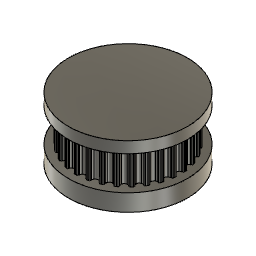
GT2 Pulley (parametric) v4 (Autodesk Fusion 360 design; units mm, degrees)
Autodesk Fusion 360 part; units mm, degrees
sketch "tooth profile" plane through (0, 0, 0) normal (0, 0, 1) x (1, 0, 0)
  circle A0 centre (0, 0) radius 9.5493 construction
  circle A1 centre (0, 0) radius 9.2953 construction
  circle A2 centre (0, 0) radius 8.5453 construction
  line L0 (0, 0) -> (0, 9.3781) construction
  line L1 (0, 0) -> (0.9895, 9.414) construction
  line L2 (0, 0) -> (1.4012, 9.4892) construction
  arc A3 (0.5539, 8.6629) -> (0.8932, 8.4985) centre (0.9512, 9.0504) ccw
  arc A4 (0.3589, 9.1498) -> (0.3788, 8.9921) centre (1.3579, 9.1956) ccw
  circle A5 centre (0, 0) radius 9.1453 construction
  arc A6 (0.3589, 9.1498) -> (0.2092, 9.2929) centre (0.2091, 9.1429) ccw
  arc A7 (0.3788, 8.9921) -> (0.5539, 8.6629) centre (1.0302, 9.1275) ccw
  arc A8 (-0.2092, 9.2929) -> (-0.3589, 9.1498) centre (-0.2091, 9.1429) ccw
  arc A9 (-0.3788, 8.9921) -> (-0.3589, 9.1498) centre (-1.3579, 9.1956) ccw
  arc A10 (-0.5539, 8.6629) -> (-0.3788, 8.9921) centre (-1.0302, 9.1275) ccw
  arc A11 (-0.8932, 8.4985) -> (-0.5539, 8.6629) centre (-0.9512, 9.0504) ccw
  arc A12 (0.8932, 8.4985) -> (-0.8932, 8.4985) centre (0, 0) ccw
  line L3 (0, 9.2953) -> (0.2092, 9.2929)
  line L4 (0, 9.2953) -> (-0.2092, 9.2929)
  circle A13 centre (0, 0) radius 8.5453
  dimension "d35" = 6
  dimension "d36" = 2.4
  dimension "d37" = 0.75
  dimension "d38" = 1.004
  dimension "d40" = 0.15
  dimension "d41" = 0.15
  dimension "d42" = 1
  dimension "d43" = 0.555
  dimension "d68" = 0.2092
  dimension "d69" = 0.6654
  dimension "d88" = 17.0906
  dimension "d89" = 17.0906
  constraint coincident A0.centre A1.centre
  constraint vertical L0
  constraint coincident A1 A4.centre
  constraint coincident L2 A4.centre
  constraint concentric A0 A5
  constraint coincident A5 A6.centre
  constraint tangent A2 A3
  constraint coincident L1 A3.centre
  constraint coincident A4.start A6.start
  constraint coincident A2 A3.end
  constraint tangent A3 A7
  constraint tangent A4 A7
  constraint symmetric L0 A3.start A10.start
  constraint symmetric L0 A3.end A11.start
  constraint symmetric L0 A3 A11
  constraint symmetric L0 A4.start A8.end
  constraint symmetric L0 A4.end A9.start
  constraint symmetric L0 A4 A9
  constraint symmetric L0 A6.end A8.start
  constraint symmetric L0 A6 A8
  constraint symmetric L0 A7 A10
  constraint tangent A4 A6
  constraint coincident L0 L3.start
  constraint coincident A1 L3.start
  constraint symmetric L0 L3.start L4.start
  constraint concentric A0 A13
  measures "d35" angle of L0 L1
  measures "d36" angle of L1 L2
  measures "d37" distance of A1 A2
  measures "d38" distance of A0 A2
  measures "d40" distance of A1 A5
  measures "d41" radius of A6
  measures "d42" radius of A4
  measures "d43" radius of A3
  measures "d68" horizontal distance of L3.start A8.start
  measures "d69" radius of A7
  measures "d88" diameter of A13
  measures "d89" diameter of A13
sketch "left flange" plane through (0, 0, 0) normal (0, 0, 1) x (1, 0, 0)
  circle A0 centre (0, 0) radius 10.5493
  dimension "d44" = 21.0986
  constraint coincident A0.centre origin
  measures "d44" diameter of A0
extrude "Extrude1" add sketch "left flange" along normal blind 11 makes body 1
extrude "Extrude2" cut sketch "left flange" along normal blind 9 bodies 1
ref_plane "WorkPlane2" through (0, 0, -2) normal (0, 0, 1) x (1, 0, 0)
sketch "right flange" plane through (0, 0, -2) normal (0, 0, 1) x (1, 0, 0)
  circle A0 centre (0, 0) radius 10.5493
  dimension "d75" = 21.0986
  constraint coincident A0.centre origin
  measures "d75" diameter of A0
extrude "Extrude11" add sketch "right flange" along normal blind 11 separate body makes body 2
extrude "Extrude12" cut 1 faces at (-1.6728, 1.987, 9) along direction (0, 0, -1) blind 6 on bodies 2 bodies 2
extrude "Extrude13" cut 1 faces at (-1.6728, 1.987, -2) along direction (0, 0, 1) blind 2 on bodies 2 bodies 2
extrude "Extrude14" add sketch "tooth profile" along normal blind 9 separate body contours A3 A4 A6 A7 A8 A9 A10 A11 A12 L3 L4 A13 makes body 3
pattern_circular "C-Pattern2" count 30 over 360 about axis through (0, 0, 1.75) along (0, 0, 1) of bodies 3 makes body 4 at (-1.0907, 8.4754, 3) makes body 5 at (-4.0993, 7.4979, 6) makes body 6 at (-5.5686, 6.4817, 6) makes body 7 at (-6.7945, 5.1823, 6) makes body 8 at (-7.4497, 4.1863, 6) makes body 9 at (-7.8853, 3.2931, 3) makes body 10 at (-8.3976, 1.5817, 3) makes body 11 at (-8.543, -0.1988, 3) makes body 12 at (-8.0958, -2.735, 6) makes body 13 at (-7.7235, -3.6564, 3) makes body 14 at (-6.7945, -5.1823, 3) makes body 15 at (-5.5686, -6.4817, 3) makes body 16 at (-4.0993, -7.4979, 3) makes body 17 at (-2.4508, -8.1863, 3) makes body 18 at (-0.6952, -8.517, 3) makes body 19 at (1.8738, -8.3373, 6) makes body 20 at (4.0993, -7.4979, 6) makes body 21 at (4.4437, -7.299, 3) makes body 22 at (6.4165, -5.6436, 6) makes body 23 at (7.0283, -4.8606, 3) makes body 24 at (7.8853, -3.2931, 3) makes body 25 at (8.3976, -1.5817, 3) makes body 26 at (8.543, 0.1988, 3) makes body 27 at (7.8853, 3.2931, 6) makes body 28 at (7.7235, 3.6564, 3) makes body 29 at (6.7945, 5.1823, 3) makes body 30 at (5.5686, 6.4817, 3) makes body 31 at (4.0993, 7.4979, 3) makes body 32 at (2.4508, 8.1863, 3)
extrude "Extrude16" add sketch "tooth profile" along normal blind 9 contours A12 A13 bodies 2 23 24 25 26 27 28 29 30 31 32 3 1 4 5 6 7 8 9 10 11 12 13 14 15 16 17 18 19 20 21 22
equation "pitch = 2 mm"
equation "shoulder_radius = 0.15 mm"
equation "transition_radius = 1.0 mm"
equation "tooth_radius = 0.555 mm"
equation "b = 0.4 mm"
equation "tooth_height = 0.75 mm"
equation "pld_to_tooth_root = 0.254 mm"
equation "flange_width_left = 2 mm"
equation "flange_height_left = 2 mm"
equation "flange_width_right = 3 mm"
equation "flange_height_right = 2 mm"
equation "tooth_count = 30"
equation "belt_width = 6 mm"
equation "tooth_angle = ( 360 / tooth_count ) * 1 deg"
equation "tooth_offset_angle = tooth_angle * ( 0.4 / 2 )"
equation "d35 = tooth_angle / 2"
equation "d36 = tooth_offset_angle"
equation "d37 = tooth_height"
equation "d38 = tooth_height + pld_to_tooth_root"
equation "d39 = ( tooth_count * pitch ) / PI"
equation "d40 = shoulder_radius"
equation "d41 = shoulder_radius"
equation "d42 = transition_radius"
equation "d43 = tooth_radius"
equation "d44 = pitch_line_diameter + flange_height_left"
equation "pitch_line_diameter = tooth_count * pitch / PI"
equation "d46 = flange_width_right + belt_width + flange_width_left"
equation "d48 = flange_width_right + belt_width"
equation "d75 = pitch_line_diameter + flange_height_right"
equation "d76 = 2 mm + flange_width_right + belt_width"
equation "d78 = -1 * belt_width"
equation "d82 = flange_width_right + belt_width"
equation "d84 = tooth_count"
equation "d88 = pitch_line_diameter - pld_to_tooth_root * 2 - tooth_height * 2"
equation "d92 = flange_width_right + belt_width"
named bodies: "left flange", "right flange", "core", "core (1)", "core (2)", "core (3)", "core (4)", "core (5)", "core (6)", "core (7)", "core (8)", "core (9)", "core (10)", "core (11)", "core (12)", "core (13)", "core (14)", "core (15)", "core (16)", "core (17)", "core (18)"
